AgriRover_Armforelink (Autodesk Fusion 360 design; units mm, degrees)
part number: 2026-09-20-16-54-42-550
Autodesk Fusion 360 part; units mm, degrees
note: some values were not read from the file. Set by a fixed rule: which sketch regions a step uses.
sketch "Sketch1" plane through (0, 0, 0) normal (0, 0, 1) x (1, 0, 0)
  line L0 (-125, 55) -> (-25, 55)
  line L1 (-25, 55) -> (-25, 30)
  line L2 (-25, 30) -> (-125, 30)
  line L3 (-125, 30) -> (-125, 55)
  circle A0 centre (-125, 42.5) radius 12.5
  circle A1 centre (-25, 42.5) radius 12.5
  dimension "d1" = 100
  dimension "d2" = 25
  constraint horizontal L0
  constraint vertical L1
  constraint horizontal L2
  constraint vertical L3
  constraint midpoint L3 A0.centre
  constraint coincident L2.end A0
  constraint midpoint L1 A1.centre
  constraint coincident L1.end A1
  measures "d1" distance of L0.start L0.end
  measures "d2" distance of L0.start L2.end
extrude "Extrude1" add sketch "Sketch1" along normal blind 30 makes body 1
sketch "Sketch2" plane through (0, 55, 0) normal (0, 1, 0) x (-1, 0, 0)
  line L0 (25, 0) -> (125, 0)
  line L1 (125, 0) -> (125, 30)
  line L2 (125, 30) -> (25, 30)
  line L3 (25, 30) -> (25, 0)
  line L4 (120, 5) -> (30, 5)
  line L5 (30, 5) -> (30, 25)
  line L6 (30, 25) -> (120, 25)
  line L7 (120, 25) -> (120, 5)
  constraint horizontal L4
  constraint vertical L5
  constraint horizontal L6
  constraint vertical L7
extrude "Extrude2" cut sketch "Sketch2" against normal blind 100 contours L4 L5 L6 L7 bodies 1
sketch "Sketch3" plane through (-120, 0, 0) normal (1, 0, 0) x (0, 1, 0)
  line L0 (30, 25) -> (30, 5)
  line L1 (30, 5) -> (55, 5)
  line L2 (55, 5) -> (55, 25)
  line L3 (55, 25) -> (30, 25)
  line L4 (55, 6) -> (30, 6)
  line L5 (30, 6) -> (30, 24)
  line L6 (30, 24) -> (55, 24)
  line L7 (55, 24) -> (55, 6)
  constraint horizontal L4
  constraint vertical L5
  constraint horizontal L6
  constraint vertical L7
  constraint coincident L0 L5.end
  constraint coincident L2 L4.start
extrude "Extrude3" cut sketch "Sketch3" against normal blind 20 contours L0 L2 L4 L5 L6 L7 bodies 1
extrude "Extrude4" cut 1 faces at (-130.9629, 42.6013, 24) along direction (0, 0, 1) blind 1 on bodies 1 bodies 1
extrude "Extrude5" cut 1 faces at (-121.6667, 46.6667, 6) along direction (0, 0, -1) blind 1 on bodies 1 bodies 1
extrude "Extrude6" cut 1 faces at (-30, 46.6667, 11.6667) along direction (1, 0, 0) blind 20 on bodies 1 bodies 1 makes body 2 at (-58.3333, 38.3333, 30)
sketch "Sketch4" plane through (0, 0, 25) normal (0, 0, -1) x (1, 0, 0)
  line L0 (-25, -30) -> (-125, -30)
  arc A0 (-125, -30) -> (-125, -55) centre (-125, -42.5) ccw
  line L1 (-125, -55) -> (-25, -55)
  arc A1 (-25, -55) -> (-25, -30) centre (-25, -42.5) ccw
  circle A2 centre (-25, -42.5) radius 12.4782
  line L2 (-37.4782, -55) -> (-37.4782, -30)
  line L3 (-37.4782, -55) -> (-47.4782, -55)
  line L4 (-47.4782, -55) -> (-47.4782, -30)
  line L5 (-47.4782, -30) -> (-37.4782, -30)
  line L6 (-37.4782, -30) -> (-37.4782, -55)
  dimension "d15" = 10
  constraint concentric A1 A2
  constraint coincident L1 L2.start
  constraint coincident L0 L2.end
  constraint perpendicular L0 L2
  constraint tangent A2 L2
  constraint horizontal L3
  constraint vertical L4
  constraint horizontal L5
  constraint vertical L6
  measures "d15" distance of L2.start L3.end
extrude "Extrude7" add sketch "Sketch4" along normal blind 25 contours L0 L1 L2 L3 L4 L5 L6 bodies 1 2
sketch "Sketch5" plane through (0, 0, 25) normal (0, 0, -1) x (1, 0, 0)
  line L0 (-47.4782, -55) -> (-47.4782, -30)
  line L1 (-47.4782, -30) -> (-125, -30)
  arc A0 (-125, -30) -> (-125, -55) centre (-125, -42.5) ccw
  line L2 (-125, -55) -> (-47.4782, -55)
  circle A1 centre (-125, -42.5) radius 12.5
  line L3 (-112.5, -55) -> (-112.5, -30)
  line L4 (-112.5, -55) -> (-102.5, -55)
  line L5 (-102.5, -55) -> (-102.5, -30)
  line L6 (-102.5, -30) -> (-112.5, -30)
  line L7 (-112.5, -30) -> (-112.5, -55)
  dimension "d18" = 10
  constraint concentric A0 A1
  constraint coincident L2 L3.start
  constraint coincident L1 L3.end
  constraint perpendicular L1 L3
  constraint tangent A1 L3
  constraint horizontal L4
  constraint vertical L5
  constraint horizontal L6
  constraint vertical L7
  measures "d18" distance of L3.start L4.end
extrude "Extrude8" add sketch "Sketch5" along normal blind 25 contours L1 L2 L3 L4 L5 L6 L7 bodies 1
sketch "Sketch6" plane through (0, 0, 0) normal (0, 0, -1) x (1, 0, 0)
  line L0 (-25, -30) -> (-125, -30)
  arc A0 (-125, -30) -> (-125, -55) centre (-125, -42.5) ccw
  line L1 (-125, -55) -> (-25, -55)
  arc A1 (-25, -55) -> (-25, -30) centre (-25, -42.5) ccw
  circle A2 centre (-25, -42.5) radius 3
  circle A3 centre (-125, -42.5) radius 3
  dimension "d21" = 6
  dimension "d22" = 6
  constraint concentric A1 A2
  constraint concentric A0 A3
  measures "d21" diameter of A2
  measures "d22" diameter of A3
extrude "Extrude9" cut sketch "Sketch6" against normal blind 100 contours A2 | A3 bodies 1
sketch "Sketch7" plane through (0, 0, 0) normal (0, 0, -1) x (1, 0, 0)
  circle A0 centre (-125, -42.5) radius 3
  circle A1 centre (-25, -42.5) radius 3
  line L0 (-25, -30) -> (-125, -30)
  arc A2 (-125, -30) -> (-125, -55) centre (-125, -42.5) ccw
  line L1 (-125, -55) -> (-25, -55)
  arc A3 (-25, -55) -> (-25, -30) centre (-25, -42.5) ccw
  line L2 (-50, -50) -> (-70, -50)
  line L3 (-70, -50) -> (-70, -36)
  line L4 (-70, -36) -> (-50, -36)
  line L5 (-50, -36) -> (-50, -50)
  line L6 (-101, -50) -> (-81, -50)
  line L7 (-81, -50) -> (-81, -36)
  line L8 (-81, -36) -> (-101, -36)
  line L9 (-101, -36) -> (-101, -50)
  dimension "d25" = 20
  dimension "d26" = 14
  constraint horizontal L2
  constraint vertical L3
  constraint horizontal L4
  constraint vertical L5
  constraint horizontal L6
  constraint vertical L7
  constraint horizontal L8
  constraint vertical L9
  measures "d25" distance of L6.start L6.end
  measures "d26" distance of L6.start L8.end
extrude "Extrude10" cut sketch "Sketch7" against normal blind 100 contours L2 L3 L4 L5 | L6 L7 L8 L9 bodies 1
fillet "Fillet1" radius 3 4 edges at (-50, 36, 2.5) (-70, 36, 2.5) (-70, 50, 2.5) (-50, 50, 2.5) on bodies 1
fillet "Fillet2" radius 3 4 edges at (-81, 50, 2.5) (-81, 36, 2.5) (-101, 36, 2.5) (-101, 50, 2.5) on bodies 1
fillet "Fillet3" radius 3 8 edges at (-70, 36, 27.5) (-101, 36, 27.5) (-81, 36, 27.5) (-50, 36, 27.5) (-50, 50, 27.5) (-81, 50, 27.5) (-70, 50, 27.5) (-101, 50, 27.5) on bodies 1
fillet "Fillet4" radius 1 tangency weight 0.61578 4 edges at (-75, 55, 30) (-137.5, 42.5, 30) (-75, 30, 30) (-12.5, 42.5, 30) on bodies 1
fillet "Fillet5" radius 1 4 edges at (-137.5, 42.5, 0) (-75, 55, 0) (-12.5, 42.5, 0) (-75, 30, 0) on bodies 1
fillet "Fillet6" radius 1 8 edges at (-37.4782, 30, 15) (-47.4782, 30, 15) (-37.4782, 55, 15) (-47.4782, 55, 15) (-102.5, 55, 15) (-102.5, 30, 15) (-112.5, 55, 15) (-112.5, 30, 15) on bodies 1
fillet "Fillet7" radius 1 4 edges at (-74.9891, 55, 5) (-74.9891, 55, 25) (-74.9891, 30, 5) (-74.9891, 30, 25) on bodies 1
